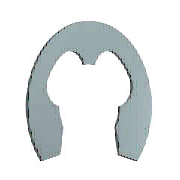
# Autodesk Inventor part: ANSI B27.7M - 3CMI-13
Saved by Autodesk Inventor 2017.3 (Build 213256000, 256)
## iProperties
IsCustomPart: 1
Created: 2016-02-22
Part Number: ANSI B27.7M - 3CMI-13
Material: Nerezová ocel
Description: Metrické pojistné kroužky se zmenšeným průřezem – vnější řada kroužků E - 3CMI
Document SubType Name: Modeling
Standard: ANSI B27.7M
Designer: Darena
Standards Organization: ANSI
Language: cs-CZ
Size Designation: 3CMI-13
Categories: <MemberInstance><Categories><Category DisplayName="Součásti hřídele" InternalName="7f7aeb1f-a693-4053-b835-cee3144e0d98" Mnemonic="SHFT"><Category DisplayName="Rozpěrné pojistné kroužky" InternalName="413b042a-1f46-4051-a560-0e0e417af91f" Mnemonic="CLIP"><CategoryParameter DisplayName="Tloušťka" InternalName="230c7f7c-2544-4c6d-b8d5-773e831b23fa" Mnemonic="thick"/><CategoryParameter DisplayName="Průměr drážky" InternalName="4054b45c-161d-4ad6-befb-f30b3855ce84" Mnemonic="grvdia"/><CategoryParameter DisplayName="Šířka drážky" InternalName="4dde6996-4bf1-443b-8317-d4f4fc6b9be0" Mnemonic="NB"/><CategoryParameter DisplayName="Průměr hřídele" InternalName="a433c9ab-b9eb-4798-a453-f2210a67728e" Mnemonic="shaftdia"/><Category DisplayName="Externí" InternalName="a9a2b132-a8be-48ab-9c3d-0c324a909558" Mnemonic="OUCLIP"><CategoryParameter DisplayName="Min. průměr hřídele" InternalName="62b77b9b-1e86-4b9a-9911-d7c0fa48fc9a" Mnemonic="shaftdiamin"/><CategoryParameter DisplayName="Vnitřní průměr" InternalName="a3599e7b-be7c-41b5-9a50-6dab253b0906" Mnemonic="outdia"/></Category></Category></Category><Category DisplayName="Typdat" InternalName="23b78d0f-2648-40c6-8793-ca6db495c9e8" Mnemonic="DATATYPE"><CategoryParameter DisplayName="Zobrazovanýnázev" InternalName="05415f3d-3907-474b-a020-eb9d644f4cf3" Mnemonic="DISPLAYNAME"/><CategoryParameter DisplayName="Norma" InternalName="0c0a119c-1e12-4c84-803f-101930972f5e" Mnemonic="STANDARD"/><CategoryParameter DisplayName="Popis" InternalName="13903e3d-64b1-4950-80da-f627842ea37f" Mnemonic="DESCRIPTION"/><CategoryParameter DisplayName="Označení" InternalName="2675968c-4ce5-49e0-a4f5-552d29089031" Mnemonic="DESIGNATION"/><CategoryParameter DisplayName="Výchozí řada" InternalName="2af9ec52-faaa-4026-b378-f9fa4afca842" Mnemonic="DEFAULTROW"/><CategoryParameter DisplayName="Název složky" InternalName="3f06958e-8713-4116-9be7-ed6184ecc97b" Mnemonic="FOLDERNAME"/><CategoryParameter DisplayName="GUID verze" InternalName="45a75005-10b1-4dfc-8d6d-dfe629f0b93c" Mnemonic="REVISIONGUID"/><CategoryParameter DisplayName="Názevsouboru" InternalName="8b46a4cc-9585-4fed-90c3-899f57e09a73" Mnemonic="FILENAME"/><CategoryParameter DisplayName="Normalizační institut" InternalName="8f5914e1-4693-403f-8ab5-d37768198c9d" Mnemonic="STDSORG"/><CategoryParameter DisplayName="Verze rodiny" InternalName="914462f6-6e19-4b14-ba84-155b9680b1d0" Mnemonic="FAMILYREVISION"/><CategoryParameter DisplayName="Revize normy" InternalName="91d5a463-65c2-4fde-b823-3b7fea5e8e17" Mnemonic="STANDARDREVISION"/><CategoryParameter DisplayName="Revize členu" InternalName="a65d44b9-392f-4f4f-857b-e4b3d54996fe" Mnemonic="MEMBERREVISION"/><CategoryParameter DisplayName="Formátoříznutí" InternalName="bc51e27b-3422-4e78-93ef-cec197ddf230" Mnemonic="CLIPFORMAT"/><CategoryParameter DisplayName="Výrobce" InternalName="cd6c7a72-a28a-4e50-99a9-2c7f4e13e5ad" Mnemonic="MANUFACTURER"/><CategoryParameter DisplayName="Internínázev" InternalName="cf1d0246-76d9-4b4a-8305-fa0409afb5c1" Mnemonic="INTERNALNAME"/><CategoryParameter DisplayName="Jemetrický" InternalName="e2385c5b-1ea4-4823-96a8-8de651266ec3" Mnemonic="ISMETRIC"/><Category DisplayName="Díl" InternalName="c0e0b642-3bcb-4cc8-9e80-f96d35c4afa4" Mnemonic="PART"><CategoryParameter DisplayName="Číslo dílu" InternalName="016b6077-bfbe-49bd-92c9-d8d59c39c941" Mnemonic="PARTNUMBER"/><CategoryParameter DisplayName="Skladové číslo" InternalName="4dba7c1c-e26c-444e-836c-b08b433409a8" Mnemonic="STOCKNUMBER"/><CategoryParameter DisplayName="Materiál pera" InternalName="5c9a8adb-dd2b-4535-b97f-0a94a95fe41f" Mnemonic="MATERIALKEY"/><CategoryParameter DisplayName="Materiál" InternalName="818a152a-d3c3-49ca-80ee-df7d91421b8e" Mnemonic="MATERIAL"/></Category></Category><Category DisplayName="Původní mapování DA" InternalName="924fff40-ddd0-4eff-ad42-30e3774ef79e" Mnemonic="LEGACYMAPDA"><CategoryParameter DisplayName="DACookie" InternalName="316934ee-8fe1-4c7a-9c36-f2d79e1add1a" Mnemonic="DACOOKIE"/></Category></Categories><FamilyTemplate Id="a2773cmi"><FamilyTemplateParameters><FamilyTemplateParameter ObjectType="kUserParameterObject" ValueType="xs:double" Id="1" ObjectReferenceKey="sd"/><FamilyTemplateParameter ObjectType="kUserParameterObject" ValueType="xs:double" Id="2" ObjectReferenceKey="Diam"/><FamilyTemplateParameter ObjectType="kUserParameterObject" ValueType="xs:double" Id="3" ObjectReferenceKey="Diam3"/><FamilyTemplateParameter ObjectType="kUserParameterObject" ValueType="xs:double" Id="4" ObjectReferenceKey="ParT"/><FamilyTemplateParameter ObjectType="kUserParameterObject" ValueType="xs:string" Id="117" ObjectReferenceKey="TEMPLATE"/><FamilyTemplateParameter ObjectType="kPropertyObject" ValueType="xs:string" Id="100" ObjectReferenceKey="{32853F0F-3444-11d1-9E93-0060B03C1CA6}" SubObjectId="52"/><FamilyTemplateParameter ObjectType="kPropertyObject" ValueType="xs:string" Id="105" ObjectReferenceKey="{32853F0F-3444-11d1-9E93-0060B03C1CA6}" SubObjectId="5"/><FamilyTemplateParameter ObjectType="kPartComponentDefinitionObject" ValueType="xs:string" Id="110" SubObjectId="Material"/></FamilyTemplateParameters></FamilyTemplate><CategoryParameterMap><ParamToTemplateMap><ParamToTemplate CategoryParameter="//CategoryParameter[@InternalName='05415f3d-3907-474b-a020-eb9d644f4cf3']" ConstantValue="ANSI B27.7M"/><ParamToTemplate CategoryParameter="//CategoryParameter[@InternalName='cf1d0246-76d9-4b4a-8305-fa0409afb5c1']" ConstantValue="ACBE07DC-D250-44DA-8DD0-24F558CF853A"/><ParamToTemplate CategoryParameter="//CategoryParameter[@InternalName='3f06958e-8713-4116-9be7-ed6184ecc97b']" ConstantValue="ANSI B27.7M"/><ParamToTemplate CategoryParameter="//CategoryParameter[@InternalName='914462f6-6e19-4b14-ba84-155b9680b1d0']" ConstantValue="10"/><ParamToTemplate CategoryParameter="//CategoryParameter[@InternalName='bc51e27b-3422-4e78-93ef-cec197ddf230']" ConstantValue="CF_INVENTOR.STDPARTS"/><ParamToTemplate CategoryParameter="//CategoryParameter[@InternalName='e2385c5b-1ea4-4823-96a8-8de651266ec3']" ConstantValue="true"/><ParamToTemplate CategoryParameter="//CategoryParameter[@InternalName='13903e3d-64b1-4950-80da-f627842ea37f']" ConstantValue="Metric Reduced Cross Section Retaining Rings - E Ring External Series - 3CMI"/><ParamToTemplate CategoryParameter="//CategoryParameter[@InternalName='8f5914e1-4693-403f-8ab5-d37768198c9d']" ConstantValue="ANSI"/><ParamToTemplate CategoryParameter="//CategoryParameter[@InternalName='0c0a119c-1e12-4c84-803f-101930972f5e']" ConstantValue="ANSI B27.7M"/><ParamToTemplate CategoryParameter="//CategoryParameter[@InternalName='cd6c7a72-a28a-4e50-99a9-2c7f4e13e5ad']" TemplateParameter="104"/><ParamToTemplate CategoryParameter="//CategoryParameter[@InternalName='91d5a463-65c2-4fde-b823-3b7fea5e8e17']" TemplateParameter="103"/><ParamToTemplate CategoryParameter="//CategoryParameter[@InternalName='45a75005-10b1-4dfc-8d6d-dfe629f0b93c']" ConstantValue="0a8ac831-bba6-4eba-88ec-23e2e60d67bb"/><ParamToTemplate CategoryParameter="//CategoryParameter[@InternalName='2af9ec52-faaa-4026-b378-f9fa4afca842']" ConstantValue="10"/><ParamToTemplate CategoryParameter="//CategoryParameter[@InternalName='8b46a4cc-9585-4fed-90c3-899f57e09a73']" ConstantValue="ANSI B27.7M - 3CMI-13"/><ParamToTemplate CategoryParameter="//CategoryParameter[@InternalName='a65d44b9-392f-4f4f-857b-e4b3d54996fe']" ConstantValue="87aa1b11-c696-4c11-9c9a-0ec1a639ce4b"/><ParamToTemplate CategoryParameter="//CategoryParameter[@InternalName='4dde6996-4bf1-443b-8317-d4f4fc6b9be0']" ConstantValue="1,2"/><ParamToTemplate CategoryParameter="//CategoryParameter[@InternalName='316934ee-8fe1-4c7a-9c36-f2d79e1add1a']" ConstantValue="*ANS~A2773CMI~3CMI-13*"/><ParamToTemplate CategoryParameter="//CategoryParameter[@InternalName='2675968c-4ce5-49e0-a4f5-552d29089031']" TemplateParameter="100"/><ParamToTemplate CategoryParameter="//CategoryParameter[@InternalName='4054b45c-161d-4ad6-befb-f30b3855ce84']" TemplateParameter="2"/><ParamToTemplate CategoryParameter="//CategoryParameter[@InternalName='818a152a-d3c3-49ca-80ee-df7d91421b8e']" TemplateParameter="110"/><ParamToTemplate CategoryParameter="//CategoryParameter[@InternalName='016b6077-bfbe-49bd-92c9-d8d59c39c941']" TemplateParameter="105"/><ParamToTemplate CategoryParameter="//CategoryParameter[@InternalName='230c7f7c-2544-4c6d-b8d5-773e831b23fa']" TemplateParameter="4"/><ParamToTemplate CategoryParameter="//CategoryParameter[@InternalName='a433c9ab-b9eb-4798-a453-f2210a67728e']" TemplateParameter="1"/></ParamToTemplateMap></CategoryParameterMap></MemberInstance>
Density: 8 g/cm^3
Appearance: Pololeštěná
Author: Darena
Autodesk Inventor part; units mm, degrees
ref_plane "YZ Plane" through (0, 0, 0) normal (1, 0, 0) x (0, 1, 0)
ref_plane "XZ Plane" through (0, 0, 0) normal (0, 1, 0) x (-1, 0, 0)
ref_plane "XY Plane" through (0, 0, 0) normal (0, 0, 1) x (1, 0, 0)
sketch "Náčrt1" plane through (0, 0, 0) normal (0, 0, 1) x (1, 0, 0)
  point P0 (0, 0)
sketch "Náčrt2" plane through (0, 0, 0) normal (0, 0, 1) x (1, 0, 0)
  line L0 (-8.0912, 0) -> (-5.15, 0)
  arc A0 (-0.9091, 8.0399) -> (-8.0912, 0) centre (0, 0) ccw
  line L1 (-0.9091, 8.0399) -> (-0.9091, 5.0691)
  arc A1 (0.9091, 5.0691) -> (-0.9091, 5.0691) centre (0, 0) ccw
  line L2 (0.9091, 5.0691) -> (0.9091, 8.0399)
  arc A2 (8.0912, 0) -> (0.9091, 8.0399) centre (0, 0) ccw
  line L3 (5.15, 0) -> (8.0912, 0)
  arc A3 (4.2917, -2.8468) -> (5.15, 0) centre (0, 0) ccw
  line L4 (4.2917, -2.8468) -> (5.075, -8.7902)
  arc A4 (5.075, -8.7902) -> (-5.075, -8.7902) centre (0, 0) ccw
  line L5 (-4.2917, -2.8468) -> (-5.075, -8.7902)
  arc A5 (-5.15, 0) -> (-4.2917, -2.8468) centre (0, 0) ccw
  line L6 (-16.1, 0) -> (16.1, 0) projected
  line L7 (0, -14.2512) -> (0, 15.7919) projected
  dimension "d1" = 0
  dimension "d3" = 5.15
  dimension "d5" = 10.15
  dimension "d7" = 0
  dimension "d9" = 8.0912
  dimension "d11" = 0.9091
  dimension "d13" = 0.9091
  dimension "d15" = 5.075
  dimension "d17" = 5.075
  dimension "d19" = 8.5833
  constraints: 12 end point, 12 point on circle, 6 centre point, 6 concentric, 2 collinear, 2 horizontal, 2 vertical, 1 equal length, 1 horizontal alignment, 1 point on line
  measures "d1" vertical distance of L0.end A1.centre
  measures "d3" radius of A1
  measures "d5" radius of A4
  measures "d7" vertical distance of L4.start L5.start
  measures "d9" radius of A2
  measures "d11" horizontal distance of L2.start A1.centre
  measures "d13" horizontal distance of L1.end A1.centre
  measures "d15" horizontal distance of L5.end A1.centre
  measures "d17" horizontal distance of L4.end A1.centre
  measures "d19" distance of L5.start L4.start
extrude "Vysunutí1" add sketch "Náčrt2" along normal blind 1.1 contours L6 A4 L7 A1 L1 A0 | L0 A5 L5 A4 L6 | A4 L6 A2 L2 A1 L7 | L3 L6 A4 L4 A3
fillet "Zaoblení1" radius 1.3273 4 edges at (-8.0912, 0, 0.55) (-0.9091, 8.0399, 0.55) (0.9091, 8.0399, 0.55) (8.0912, 0, 0.55)
chamfer "Zkosení1" distance 1.015 distance2 1.6222 1 edges at (-5.075, -8.7902, 0.55) measured on face at (-4.4798, 9.1079, 0.7333)
chamfer "Zkosení2" distance 1.6222 distance2 1.015 1 edges at (5.075, -8.7902, 0.55) measured on face at (4.8139, -6.809, 0.3667)
equation "\"d3\" = 0.5 * Diam"
equation "\"d5\" = 0.5 * Diam3"
equation "\"d9\" = 0.294118 * Diam3 + 0.205882 * Diam"
equation "\"d11\" = 0.0909091 * Diam3 - 0.0909091 * Diam"
equation "\"d13\" = 0.0909091 * Diam3 - 0.0909091 * Diam"
equation "\"d15\" = 0.25 * Diam3"
equation "\"d17\" = 0.25 * Diam3"
equation "\"d19\" = 0.833333 * Diam"
equation "\"d20\" = ParT"
equation "\"d22\" = 0.181818 * Diam3 - 0.181818 * sd"
equation "\"d23\" = 0.05 * Diam3"
equation "\"d24\" = 0.222222 * Diam3 - 0.222222 * sd"
equation "\"d25\" = 0.222222 * Diam3 - 0.222222 * sd"
equation "\"d26\" = 0.05 * Diam3"
equation "\"Diam3\" = 20.3"
equation "\"ParT\" = 1.1"
equation "\"Diam\" = 10.3"
equation "\"sd\" = 13"
equation "\"TEMPLATE\" = 1.2345"
body "Solid1"
